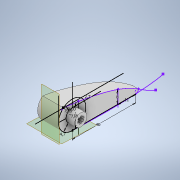
# Autodesk Inventor part: rachag5
Saved by Autodesk Inventor 2020 (Build 240168000, 168)
## iProperties
Created: 2023-10-21
Part Number: rachag5
Material: Типовые
Document SubType Name: Modeling
Designer: 522
Density: 1 g/cm^3
Appearance: По умолчанию
Author: 522
Autodesk Inventor part; units mm, degrees
ref_plane "YZ Plane" through (0, 0, 0) normal (1, 0, 0) x (0, 1, 0)
ref_plane "XZ Plane" through (0, 0, 0) normal (0, 1, 0) x (-1, 0, 0)
ref_plane "XY Plane" through (0, 0, 0) normal (0, 0, 1) x (1, 0, 0)
sketch "Эскиз1" plane through (0, 0, 0) normal (1, 0, 0) x (0, 1, 0)
  circle A0 centre (0, 0) radius 3.85
  circle A1 centre (0, 0) radius 8.55
  line L0 (-8.55, 0) -> (-8.55, -40)
  line L1 (6.55, 5.6577) -> (6.55, -32.1821)
  line L2 (3.85, 0) -> (3.85, -17.9751)
  line L3 (0, 0) -> (14.53, 0)
  line L4 (0, 0) -> (0, 8.55)
  line L5 (14.53, 8.55) -> (0, 8.55)
  arc A2 (-8.55, -39.75) -> (-6.7329, -41.4987) centre (-6.8, -39.75) ccw
  line L6 (6.55, 1.7425) -> (6.55, 23.1247)
  line L7 (0, 0) -> (17.6875, 0)
  line L8 (0, 0) -> (6.7983, 3.925)
  line L9 (0, 0) -> (7.85, 0) construction
  spline S0 degree 2 poles (-8.55, 0) (-10.1106, -39.8429) (-6.4852, -57.0244) knots 0 0 0 1 1 1
  line L10 (-8.55, -39.75) -> (-8.55, -28.75)
  line L11 (-8.55, -28.75) -> (-3.0195, -28.75)
  line L12 (-8.55, -28.75) -> (-0.55, -28.75)
  line L13 (0, -3.85) -> (-12.7006, -3.85)
  line L14 (-8.6905, -3.85) -> (5.3095, -3.85)
  spline S1 degree 4 poles (6.55, 5.4955) (6.3518, 3.1029) (1.3238, -41.696) (-6.4796, -36.4642) (-12.7006, -52.3006) knots 0 0 0 0 0 1 1 1 1 1
  line L15 (-8.55, -28.75) -> (-9.1038, -28.75)
  line L16 (-8.5374, -28.75) -> (-10.4405, -28.75)
  point P0 (5.9063, 6.1821)
  point P1 (-8.55, -39.75)
  point P2 (3.85, -7.6341)
  point P3 (-8.5374, -39.9594)
  dimension "d0" = 7.7
  dimension "d1" = 4.7
  dimension "d4" = 2.7
  dimension "d100" = 40
  dimension "d141" = 7.85
  dimension "d142" = 30
  dimension "d143" = 11
  dimension "d144" = 8
  dimension "d145" = 14
  constraints: 34 end point, 9 point on line, 8 point on circle, 5 horizontal, 5 vertical, 4 tangent, 3 centre point, 2 coincident, 2 perpendicular, 1 equal length, 9 other
  measures "d0" diameter of A0
  measures "d1" radial gap between concentric circles of A1 A0
  measures "d4" distance between parallel lines of L2 L1
  measures "d100" distance of L0.start L0.end
  measures "d141" distance of L3.start L8.end
  measures "d142" angle of L9 L8
  measures "d143" distance of L10.start L10.end
  measures "d144" distance of L10.end L12.end
  measures "d145" distance of L14.start L14.end
extrude "Выдавливание1" add sketch "Эскиз1" against normal blind 13 contours A0 L4 L3 | L13 A1 L4 A0 | L14 L2 A1 L13 | A0 L2 L14 | L3 L8 A0 | L3 S1 L14 L2 | A0 L8 S1 L3 | L4 A1 S1 L8 A0 | A0 L8 L4 | L13 L0 A1 | A1 L2 S1 L12 L11 L0 L13 | L14 S1 A1 L2 | L0 L13 S0 | A1 S1 L2 | L0 L15 S0 L13 | L11 L12 S1 A2 S0 L0 | L0 S0 L15
sketch "Эскиз2" plane through (0, 0, 0) normal (1, 0, 0) x (0, 0, -1)
  line L0 (0, 0) -> (0, 14.4854)
  line L1 (0, 14.4854) -> (-8.5902, 14.4854)
  line L2 (-8.5902, 14.4854) -> (-8.55, -0.0237)
  arc A0 (-5.4955, 6.55) -> (0, -8.55) centre (0, 0) ccw projected
  point P0 (0, 8.55)
  point P1 (0, 8.55)
  point P2 (0, 8.55)
  point P3 (0, 8.55)
  point P4 (0, 8.55)
  point P5 (0, 8.55)
  point P6 (0, 8.55)
  point P7 (0, 8.55)
  point P8 (0, 8.55)
  constraints: 6 end point, 1 perpendicular, 1 point on circle, 1 tangent, 1 vertical
ref_plane "РабПлоскость1" through (0, 14.53, 8.55) normal (0, 0, -1) x (-1, 0, 0)
sketch "Эскиз5" plane through (0, 0, 0) normal (1, 0, 0) x (0, 0, -1)
  circle A0 centre (0, 0) radius 3.85
  line L0 (-11.3638, -1.8204) -> (-10.1238, -1.8204)
  line L1 (-10.1238, -1.8204) -> (-10.1238, -2.8204)
  line L2 (-10.1238, -2.8204) -> (-11.3638, -2.8204)
  line L3 (-11.3638, -2.8204) -> (-11.3638, -1.8204)
  line L4 (-11.3638, -1.8204) -> (-10.1238, -2.8204) construction
  line L5 (-10.1238, -1.8204) -> (-11.3638, -2.8204) construction
  line L6 (-10.6834, -1.8204) -> (-10.1238, -2.1204)
  line L7 (-10.6834, -2.8204) -> (-10.1238, -2.5204)
  circle A1 centre (0, 0) radius 2.1
  circle A2 centre (0, 0) radius 1.5
  line L8 (-2.7458, -0.0236) -> (-2.5722, 0.9613)
  line L9 (-2.5722, 0.9613) -> (-1.3904, 0.7529)
  line L10 (-1.3904, 0.7529) -> (-1.564, -0.2319)
  line L11 (-1.564, -0.2319) -> (-2.7458, -0.0236)
  line L12 (-2.7458, -0.0236) -> (-1.3904, 0.7529) construction
  line L13 (-2.5722, 0.9613) -> (-1.564, -0.2319) construction
  line L14 (-1.9218, 0.8466) -> (-1.4425, 0.4574)
  line L15 (-2.0954, -0.1382) -> (-1.5119, 0.0635)
  line L16 (-0.5812, -1.4705) -> (-1.3525, -2.3897)
  line L17 (-0.928, -1.8838) -> (-0.811, -1.2776)
  line L18 (-1.3525, -2.3897) -> (-2.1185, -1.7469)
  line L19 (-2.1185, -1.7469) -> (-0.5812, -1.4705) construction
  line L20 (-1.6941, -1.241) -> (-1.1174, -1.0205)
  line L21 (-1.3472, -0.8277) -> (-0.5812, -1.4705)
  line L22 (-1.3525, -2.3897) -> (-1.3472, -0.8277) construction
  line L23 (-2.1185, -1.7469) -> (-1.3472, -0.8277)
  line L24 (0.9829, -1.2385) -> (1.3933, -2.3662)
  line L25 (1.1674, -1.7456) -> (0.701, -1.3411)
  line L26 (1.3933, -2.3662) -> (0.4536, -2.7082)
  line L27 (0.4536, -2.7082) -> (0.9829, -1.2385) construction
  line L28 (0.2277, -2.0876) -> (0.3251, -1.4779)
  line L29 (0.0432, -1.5805) -> (0.9829, -1.2385)
  line L30 (1.3933, -2.3662) -> (0.0432, -1.5805) construction
  line L31 (0.4536, -2.7082) -> (0.0432, -1.5805)
  line L32 (1.564, 0.2319) -> (2.7458, 0.0236)
  line L33 (2.0954, 0.1382) -> (1.5119, -0.0635)
  line L34 (2.7458, 0.0236) -> (2.5722, -0.9613)
  line L35 (2.5722, -0.9613) -> (1.564, 0.2319) construction
  line L36 (1.9218, -0.8466) -> (1.4425, -0.4574)
  line L37 (1.3904, -0.7529) -> (1.564, 0.2319)
  line L38 (2.7458, 0.0236) -> (1.3904, -0.7529) construction
  line L39 (2.5722, -0.9613) -> (1.3904, -0.7529)
  line L40 (0.5812, 1.4705) -> (1.3525, 2.3897)
  line L41 (0.928, 1.8838) -> (0.811, 1.2776)
  line L42 (1.3525, 2.3897) -> (2.1185, 1.7469)
  line L43 (2.1185, 1.7469) -> (0.5812, 1.4705) construction
  line L44 (1.6941, 1.241) -> (1.1174, 1.0205)
  line L45 (1.3472, 0.8277) -> (0.5812, 1.4705)
  line L46 (1.3525, 2.3897) -> (1.3472, 0.8277) construction
  line L47 (2.1185, 1.7469) -> (1.3472, 0.8277)
  line L48 (-0.9829, 1.2385) -> (-1.3933, 2.3662)
  line L49 (-1.1674, 1.7456) -> (-0.701, 1.3411)
  line L50 (-1.3933, 2.3662) -> (-0.4536, 2.7082)
  line L51 (-0.4536, 2.7082) -> (-0.9829, 1.2385) construction
  line L52 (-0.2277, 2.0876) -> (-0.3251, 1.4779)
  line L53 (-0.0432, 1.5805) -> (-0.9829, 1.2385)
  line L54 (-1.3933, 2.3662) -> (-0.0432, 1.5805) construction
  line L55 (-0.4536, 2.7082) -> (-0.0432, 1.5805)
  point P0 (-10.7438, -2.3204)
  point P1 (-2.0681, 0.3647)
  point P2 (-1.3499, -1.6087)
  point P3 (0.7182, -1.9734)
  point P4 (2.0681, -0.3647)
  point P5 (1.3499, 1.6087)
  point P6 (-0.7182, 1.9734)
  point P7 (-1.9218, 0.8466)
  point P8 (-1.1674, 1.7456)
  point P9 (-0.2277, 2.0876)
  point P10 (0.928, 1.8838)
  point P11 (1.6941, 1.241)
  point P12 (2.0954, 0.1382)
  point P13 (1.9218, -0.8466)
  point P14 (1.1674, -1.7456)
  point P15 (0.2277, -2.0876)
  point P16 (-0.928, -1.8838)
  point P17 (-1.6941, -1.241)
  point P18 (-2.0954, -0.1382)
  point P19 (-0.928, -1.8838)
  point P20 (-1.6941, -1.241)
  dimension "d17" = 7.7
  dimension "d18" = 1
  dimension "d19" = 0.3
  dimension "d20" = 0.3
  dimension "d21" = 0.62
  dimension "d22" = 4.2
  dimension "d23" = 3
  dimension "d24" = 1
  dimension "d25" = 0.3
  dimension "d26" = 0.3
  dimension "d29" = 360
  constraints: 112 end point, 28 point on line, 14 midpoint, 4 parallel, 3 centre point, 3 coincident, 2 perpendicular, 1 horizontal, 103 other
  measures "d17" diameter of A0
  measures "d18" distance between parallel lines of L2 L0
  measures "d19" distance from line of L2 L7.end
  measures "d20" distance from line of L6.end L0
  measures "d21" distance from line of point (-10.744, -2.32) L1
  measures "d22" diameter of A1
  measures "d23" diameter of A2
  measures "d24" distance of L8.start L8.end
  measures "d25" distance of L9.end L14.end
  measures "d26" distance of L15.end L10.end
extrude "Выдавливание4" add sketch "Эскиз5" along normal blind 5.5 contours A0 | A1 L36 L37 L33 | A1 L32 L34 L39 | L44 L45 L41 A1 | A1 L40 L42 L47 | L24 L26 L31 A1 | A1 L28 L29 L25 | L52 L53 L49 A1 | A1 L48 L50 L55 | L16 L18 L23 A1 | A1 L20 L21 L17 | L14 L10 L15 A1 | A1 L11 L8 L9
extrude "Выдавливание5" cut sketch "Эскиз5" against normal blind 5 contours L32 L37 A2 L45 L47 A1 | L33 L37 L32 | L39 L37 L36 | A1 L24 L29 A2 L37 L39 | L47 L45 L44 | L25 L29 L24 | L40 L45 A2 L53 L55 A1 | L41 L45 L40 | A2 | L31 L29 L28 | A1 L16 L21 A2 L29 L31 | L55 L53 L52 | L16 L18 L23 A1 | L17 L21 L16 | L48 L53 A2 L10 L9 A1 | L49 L53 L48 | L21 L23 A1 L11 L10 A2 | L23 L21 L20 | L9 L10 L14 | L15 L10 L11
ref_plane "РабПлоскость2" through (-6.5, -8.55, 0) normal (0, -0.9992338, 0.039138) x (1, 0, 0)
sketch "Эскиз23" plane through (-6.5, -8.55, 0) normal (0, -0.9992338, 0.039138) x (1, 0, 0)
  line L0 (6.5, 8.8846) -> (-6.5, 8.8846) projected
  line L1 (-6.5, -39.9283) -> (-6.5, -41.4011) projected
  line L2 (6.5, 8.8846) -> (-6.5, 8.8846)
  line L3 (-6.5, 8.8846) -> (-6.5, -41.4011)
  line L4 (-6.5, -41.4011) -> (6.5, -41.4011)
  line L5 (6.5, -41.4011) -> (6.5, 8.8846)
  line L6 (6.5, 4.1846) -> (6.5, -3.5154) projected
  line L7 (6.5, -3.5154) -> (-5.5, -3.5154)
  line L8 (6.5, -28.775) -> (-1.5, -28.775)
  line L9 (6.5, -41.541) -> (3, -41.541)
  line L10 (-6.5, -41.4011) -> (6.5, -41.4011)
  line L11 (6.5, -41.4011) -> (6.5, -41.541)
  line L12 (6.5, -41.541) -> (-6.5, -41.541)
  line L13 (-6.5, -41.541) -> (-6.5, -41.4011)
  line L14 (-6.5, 8.8846) -> (-6.5, 0) projected
  spline S0 degree 2 poles (-6.5, 8.8846) (-5.8365, -3.5748) (-5.2186, -4.5358) knots 0 0 0 1 1 1
  spline S1 degree 4 poles (-5.8003, -1.1837) (-3.5482, -19.1397) (1.4408, -47.7835) (-1.7357, -37.5062) (26.5342, -65.5265) knots 0.16899 0.16899 0.16899 0.16899 0.16899 1 1 1 1 1
  line L15 (-6.8028, 6.8092) -> (-4.7978, -9.1765) construction
  arc A0 (-6.5368, 5.2175) -> (-4.9331, -7.5684) centre (306.9007, 38.0365) ccw construction
  point P0 (6.5, 0.3346)
  point P1 (-6.5, -41.3958)
  point P2 (-6.5, 6.0822)
  point P3 (26.5342, -65.5265)
  point P4 (-5.5, -3.5154)
  point P5 (3, -41.541)
  dimension "d146" = 12
  dimension "d148" = 8
  dimension "d149" = 3.5
  constraints: 24 end point, 4 horizontal, 4 parallel, 3 perpendicular, 2 midpoint, 2 point on line, 1 centre point, 1 point on circle, 12 other
  measures "d146" distance of L6.end L7.end
  measures "d148" distance of L8.start L8.end
  measures "d149" distance of L9.start L9.end
extrude "Выдавливание16" cut sketch "Эскиз23" against normal mid plane 33.5 contours S0 S1 L4 L1 L3 | L4 S1 L12 L13
equation "\"d19\" = d20"
equation "\"d26\" = d25"
